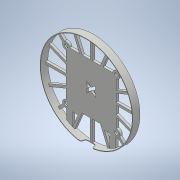
# Autodesk Inventor part: Чаша1
Saved by Autodesk Inventor 2020 (Build 240168000, 168)
## iProperties
Created: 2021-05-28
Part Number: Чаша1
Material: Типовые
Document SubType Name: Modeling
Designer: I_Love_U_Bogdan
Density: 1 g/cm^3
Appearance: По умолчанию
Author: I_Love_U_Bogdan
Autodesk Inventor part; units mm, degrees
ref_plane "YZ Plane" through (0, 0, 0) normal (1, 0, 0) x (0, 1, 0)
ref_plane "XZ Plane" through (0, 0, 0) normal (0, 1, 0) x (-1, 0, 0)
ref_plane "XY Plane" through (0, 0, 0) normal (0, 0, 1) x (1, 0, 0)
sketch "Эскиз1" plane through (0, 0, 0) normal (0, 0, 1) x (1, 0, 0)
  line L0 (7.05, 4.17398) -> (7.05, 6.642805)
  line L1 (7.05, 6.642805) -> (-5.95, -2.765587)
  line L2 (-5.95, -2.765587) -> (-5.95, 18.64843)
  line L3 (-5.95, 18.64843) -> (7.05, 9.240038)
  line L4 (7.05, 9.240038) -> (7.05, 11.708863)
  line L5 (7.05, 11.708863) -> (-4.244357, 19.882843)
  line L6 (-4.244357, 19.882843) -> (25.344357, 19.882843)
  line L7 (14.05, 11.708863) -> (25.344357, 19.882843)
  line L8 (14.05, 11.708863) -> (14.05, 9.240038)
  line L9 (27.05, 18.64843) -> (14.05, 9.240038)
  line L10 (27.05, -2.765587) -> (27.05, 18.64843)
  line L11 (14.05, 6.642805) -> (27.05, -2.765587)
  line L12 (14.05, 6.642805) -> (14.05, 4.17398)
  line L13 (25.344357, -4) -> (14.05, 4.17398)
  line L14 (-4.244357, -4) -> (25.344357, -4)
  line L15 (-4.244357, -4) -> (7.05, 4.17398)
  line L16 (-5.95, -6) -> (27.05, -6)
  line L17 (27.05, -32) -> (27.05, -6)
  line L18 (29.55, -33.117157) -> (29.55, -35)
  line L19 (31.65, -33.117157) -> (29.55, -33.117157)
  line L20 (31.65, -31.117157) -> (31.65, -33.117157)
  line L21 (29.55, -31.117157) -> (31.65, -31.117157)
  line L22 (29.55, -20.7) -> (29.55, -31.117157)
  line L23 (31.55, -20.7) -> (29.55, -20.7)
  line L24 (31.55, -19.7) -> (31.55, -20.7)
  line L25 (29.55, -16.235898) -> (31.55, -19.7)
  line L26 (29.55, 32) -> (29.55, 21.882843)
  line L27 (31.55, 19.882843) -> (29.55, 19.882843)
  line L28 (31.55, 19.882843) -> (31.55, 21.882843)
  line L29 (29.55, 21.882843) -> (31.55, 21.882843)
  line L30 (29.55, 32) -> (27.05, 32)
  line L31 (27.05, 21.882843) -> (27.05, 32)
  line L32 (-5.95, 21.882843) -> (27.05, 21.882843)
  line L33 (-5.95, 21.882843) -> (-5.95, 32)
  line L34 (-8.45, 32) -> (-5.95, 32)
  line L35 (-8.45, 32) -> (-8.45, 21.882843)
  line L36 (-8.45, 21.882843) -> (-10.45, 21.882843)
  line L37 (-10.45, 19.882843) -> (-10.45, 21.882843)
  line L38 (-10.45, 19.882843) -> (-8.45, 19.882843)
  line L39 (-8.45, -20.7) -> (-8.45, -31.117157)
  line L40 (-8.45, -16.235898) -> (-10.45, -19.7)
  line L41 (-10.45, -19.7) -> (-10.45, -20.7)
  line L42 (-10.45, -20.7) -> (-8.45, -20.7)
  line L43 (-8.45, -31.117157) -> (-10.55, -31.117157)
  line L44 (-10.55, -31.117157) -> (-10.55, -33.117157)
  line L45 (-10.55, -33.117157) -> (-8.45, -33.117157)
  line L46 (-8.45, -33.117157) -> (-8.45, -35)
  line L47 (-5.95, -32) -> (-5.95, -6)
  line L48 (10.55, 6.707009) -> (10.55, 9.175834)
  circle A0 centre (10.55, 7.941421) radius 38.2
  circle A1 centre (10.55, 7.941421) radius 38.7
  line L49 (27.05, -32) -> (27.026915, -32)
  line L50 (27.026915, -35) -> (27.026915, -32)
  line L51 (27.026915, -35) -> (29.55, -35)
  line L52 (29.55, 19.882843) -> (29.55, -16.235898)
  line L53 (-8.45, 19.882843) -> (-8.45, -16.235898)
  line L54 (-5.926915, -35) -> (-8.45, -35)
  line L55 (-5.926915, -35) -> (-5.926915, -32)
  line L56 (-5.95, -32) -> (-5.926915, -32)
  line L57 (13.55, 6.38746) -> (13.55, 5.153048)
  line L58 (11.402822, 7.941421) -> (13.55, 6.38746)
  line L59 (13.55, 9.495383) -> (11.402822, 7.941421)
  line L60 (13.55, 10.729795) -> (13.55, 9.495383)
  line L61 (10.55, 8.558628) -> (13.55, 10.729795)
  line L62 (7.55, 10.729795) -> (10.55, 8.558628)
  line L63 (7.55, 9.495383) -> (7.55, 10.729795)
  line L64 (9.697178, 7.941421) -> (7.55, 9.495383)
  line L65 (7.55, 6.38746) -> (9.697178, 7.941421)
  line L66 (7.55, 5.153048) -> (7.55, 6.38746)
  line L67 (10.55, 7.324215) -> (7.55, 5.153048)
  line L68 (13.55, 5.153048) -> (10.55, 7.324215)
  line L69 (-10.45, 28.941421) -> (31.55, 28.941421)
  line L70 (31.55, 28.941421) -> (31.55, -13.058579)
  line L71 (31.55, -13.058579) -> (-10.45, -13.058579)
  line L72 (-10.45, -13.058579) -> (-10.45, 28.941421)
  line L73 (-10.45, 28.941421) -> (31.55, -13.058579) construction
  line L74 (31.55, 28.941421) -> (-10.45, -13.058579) construction
  circle A2 centre (31.55, 28.941421) radius 1.5
  circle A3 centre (31.55, -13.058579) radius 1.5
  circle A4 centre (-10.45, -13.058579) radius 1.5
  circle A5 centre (-10.45, -13.058579) radius 3
  circle A6 centre (31.55, -13.058579) radius 3
  circle A7 centre (31.55, 28.941421) radius 3
  line L75 (34.55, 28.941421) -> (34.55, -13.058579)
  line L76 (31.55, -16.058579) -> (-10.45, -16.058579)
  line L77 (-13.45, -13.058579) -> (-13.45, 29.004231)
  line L78 (-10.391298, 31.941421) -> (31.55, 31.941421)
  circle A8 centre (-10.45, 28.941421) radius 1.5
  circle A9 centre (-10.45, 28.941421) radius 3
  line L79 (6.85, 9.1379) -> (6.85, 12.10049)
  line L80 (6.85, 12.10049) -> (10.55, 9.422716)
  line L81 (10.55, 9.422716) -> (14.25, 12.10049)
  line L82 (14.25, 12.10049) -> (14.25, 9.1379)
  line L83 (14.25, 9.1379) -> (12.596772, 7.941421)
  line L84 (12.596772, 7.941421) -> (14.25, 6.744943)
  line L85 (14.25, 6.744943) -> (14.25, 3.782353)
  line L86 (14.25, 3.782353) -> (10.55, 6.460126)
  line L87 (10.55, 6.460126) -> (6.85, 3.782353)
  line L88 (6.85, 3.782353) -> (6.85, 6.744943)
  line L89 (6.85, 6.744943) -> (8.503228, 7.941421)
  line L90 (8.503228, 7.941421) -> (6.85, 9.1379)
  line L91 (10.55, 7.941421) -> (10.55, 46.141421) construction
  line L92 (11.55, 28.941421) -> (11.55, 46.141421)
  line L93 (9.55, 46.141421) -> (9.55, 28.941421)
  line L94 (9.55, 9.28235) -> (9.55, 8.941421)
  line L95 (9.55, 8.047938) -> (9.55, 7.941421)
  line L96 (11.55, 7.941421) -> (11.55, 8.047938)
  line L97 (11.55, 8.941421) -> (11.55, 9.28235)
  line L98 (3.437527, 27.725575) -> (-3.144628, 43.616303)
  line L99 (-4.992387, 42.850936) -> (1.589768, 26.960208)
  line L100 (-3.592136, 23.497771) -> (-15.754372, 35.660007)
  line L101 (-17.168586, 34.245794) -> (-5.006349, 22.083557)
  line L102 (-8.468787, 16.901653) -> (-24.359515, 23.483808)
  line L103 (-25.124882, 21.636049) -> (-9.234154, 15.053894)
  line L104 (-10.45, 8.941421) -> (-27.65, 8.941421)
  line L105 (-27.65, 6.941421) -> (-10.45, 6.941421)
  line L106 (-9.234154, 0.828949) -> (-25.124882, -5.753206)
  line L107 (-24.359515, -7.600965) -> (-8.468787, -1.01881)
  line L108 (-5.006349, -6.200714) -> (-17.168586, -18.362951)
  line L109 (-15.754372, -19.777164) -> (-3.592136, -7.614928)
  line L110 (1.589768, -11.077365) -> (-4.992387, -26.968093)
  line L111 (-3.144628, -27.73346) -> (3.437527, -11.842732)
  line L112 (9.55, -13.058579) -> (9.55, -30.258579)
  line L113 (11.55, -30.258579) -> (11.55, -13.058579)
  line L114 (17.662473, -11.842732) -> (24.244628, -27.73346)
  line L115 (26.092387, -26.968093) -> (19.510232, -11.077365)
  line L116 (24.692136, -7.614928) -> (36.854372, -19.777164)
  line L117 (38.268586, -18.362951) -> (26.106349, -6.200714)
  line L118 (29.568787, -1.01881) -> (45.459515, -7.600965)
  line L119 (46.224882, -5.753206) -> (30.334154, 0.828949)
  line L120 (31.55, 6.941421) -> (48.75, 6.941421)
  line L121 (48.75, 8.941421) -> (31.55, 8.941421)
  line L122 (30.334154, 15.053894) -> (46.224882, 21.636049)
  line L123 (45.459515, 23.483808) -> (29.568787, 16.901653)
  line L124 (26.106349, 22.083557) -> (38.268586, 34.245794)
  line L125 (36.854372, 35.660007) -> (24.692136, 23.497771)
  line L126 (19.510232, 26.960208) -> (26.092387, 42.850936)
  line L127 (24.244628, 43.616303) -> (17.662473, 27.725575)
  line L128 (-4.992387, -16.058579) -> (-9.992387, -16.058579)
  line L129 (-9.992387, -16.058579) -> (-9.992387, -24.85645)
  line L130 (-9.992387, -27.058579) -> (-4.992387, -27.058579)
  line L131 (-4.992387, -27.058579) -> (-4.992387, -16.058579)
  line L132 (31.092387, -16.058579) -> (31.092387, -24.85645)
  line L133 (26.092387, -27.058579) -> (26.092387, -16.058579)
  point P0 (0, 0)
  point P1 (10.55, 27.041421)
  point P2 (-10.45, 15.557514)
  point P3 (-27.636909, 8.941421)
  point P4 (-25.112787, 21.631039)
  point P5 (2.933907, 28.941421)
  point P6 (-3.139618, 43.604208)
  point P7 (9.55, 46.12833)
  point P8 (34.257107, -14.351472)
  point P9 (31.55, -10.058579)
  point P10 (31.55, -1.839456)
  point P11 (45.44742, -7.595955)
  point P12 (38.259329, -18.353694)
  point P13 (0.769123, 28.941421)
  point P14 (-7.45, 28.941421)
  point P15 (-11.742893, 31.648528)
  point P16 (-15.745115, 35.65075)
  point P17 (-4.987377, 42.838841)
  point P18 (-10.45, 17.722298)
  point P19 (-24.34742, 23.478798)
  point P20 (-17.159329, 34.236537)
  point P21 (-13.157107, 30.234315)
  point P22 (-10.45, 25.941421)
  point P23 (-0.473518, -16.058579)
  point P24 (2.933907, -13.058579)
  point P25 (9.55, -30.245487)
  point P26 (-3.139618, -27.721365)
  point P27 (18.166093, -13.058579)
  point P28 (24.239618, -27.721365)
  point P29 (11.55, -30.245487)
  point P30 (21.573518, -16.058579)
  point P31 (32.842893, 31.648528)
  point P32 (28.55, 28.941421)
  point P33 (20.330877, 28.941421)
  point P34 (26.087377, 42.838841)
  point P35 (36.845115, 35.65075)
  point P36 (31.55, 17.722298)
  point P37 (31.55, 25.941421)
  point P38 (34.257107, 30.234315)
  point P39 (38.259329, 34.236537)
  point P40 (45.44742, 23.478798)
  point P41 (31.55, 15.557514)
  point P42 (46.212787, 21.631039)
  point P43 (48.736909, 8.941421)
  point P44 (31.55, 0.325329)
  point P45 (48.736909, 6.941421)
  point P46 (46.212787, -5.748196)
  point P47 (32.842893, -15.765685)
  point P48 (36.845115, -19.767908)
  point P49 (31.092387, -24.26495)
  point P50 (-5.963328, -27.058579)
  point P51 (-5.95, -27.058579)
  point P52 (-5.95, -27.064864)
  point P53 (-11.742893, -15.765685)
  point P54 (-9.992387, -24.26495)
  point P55 (-15.745115, -19.767908)
  point P56 (-10.45, -1.839456)
  point P57 (-10.45, -10.058579)
  point P58 (-13.157107, -14.351472)
  point P59 (-17.159329, -18.353694)
  point P60 (-24.34742, -7.595955)
  point P61 (-10.45, 0.325329)
  point P62 (-25.112787, -5.748196)
  point P63 (-27.636909, 6.941421)
  point P64 (11.55, 46.12833)
  point P65 (24.239618, 43.604208)
  point P66 (18.166093, 28.941421)
  dimension "d0" = 76.4
  dimension "d1" = 0.5
  dimension "d15" = 42
  dimension "d16" = 42
  dimension "d17" = 3
  dimension "d18" = 3
  dimension "d19" = 3
  dimension "d22" = 6
  dimension "d23" = 6
  dimension "d24" = 6
  dimension "d25" = 3
  dimension "d26" = 1.5
  dimension "d27" = 0.7
  dimension "d31" = 360
  dimension "d33" = 5
  dimension "d34" = 11
  constraints: 134 end point, 13 parallel, 9 point on line, 8 centre point, 8 coincident, 7 tangent, 6 point on circle, 4 midpoint, 4 symmetric about line, 3 perpendicular, 2 horizontal, 2 vertical, 114 other
  measures "d15" distance of L70.end L71.end
  measures "d16" distance of L69.end L70.end
  measures "d17" diameter of A2
  measures "d18" diameter of A3
  measures "d19" diameter of A4
  measures "d22" diameter of A5
  measures "d23" diameter of A6
  measures "d24" diameter of A7
  measures "d25" diameter of A8
  measures "d26" radial gap between concentric circles of A8 A9
  measures "d27" distance between parallel lines of L64 L90
  measures "d33" distance of L130.end L130.start
  measures "d34" distance of L130.start L128.end
sketch "Эскиз1 outline for Выдавливание1" plane through (0, 0, 0) normal (0, 0, 1) x (1, 0, 0)
  arc A0 (-5.95, -27.064864) -> (-5.963328, -27.058579) centre (10.55, 7.941421) ccw
  arc A1 (-5.963328, -27.058579) -> (-5.95, -27.064864) centre (10.55, 7.941421) ccw
  arc A2 (-11.742893, -15.765685) -> (-10.45, -16.058579) centre (-10.45, -13.058579) ccw
  line L0 (-10.45, -16.058579) -> (-9.992387, -16.058579)
  line L1 (-9.992387, -16.058579) -> (-9.992387, -24.26495)
  arc A3 (-9.992387, -24.26495) -> (-15.745115, -19.767908) centre (10.55, 7.941421) cw
  line L2 (-15.745115, -19.767908) -> (-11.742893, -15.765685)
  circle A4 centre (-10.45, -13.058579) radius 1.5
  line L3 (-4.992387, -26.968093) -> (-4.992387, -16.058579)
  line L4 (-4.992387, -16.058579) -> (-0.473518, -16.058579)
  line L5 (-0.473518, -16.058579) -> (-4.992387, -26.968093)
  line L6 (-3.139618, -27.721365) -> (2.933907, -13.058579)
  line L7 (2.933907, -13.058579) -> (9.55, -13.058579)
  line L8 (9.55, -13.058579) -> (9.55, -30.245487)
  arc A5 (9.55, -30.245487) -> (-3.139618, -27.721365) centre (10.55, 7.941421) cw
  line L9 (-24.34742, -7.595955) -> (-10.45, -1.839456)
  line L10 (-10.45, -1.839456) -> (-10.45, -10.058579)
  arc A6 (-10.45, -10.058579) -> (-13.157107, -14.351472) centre (-10.45, -13.058579) ccw
  line L11 (-13.157107, -14.351472) -> (-17.159329, -18.353694)
  arc A7 (-17.159329, -18.353694) -> (-24.34742, -7.595955) centre (10.55, 7.941421) cw
  line L12 (-27.636909, 6.941421) -> (-10.45, 6.941421)
  line L13 (-10.45, 6.941421) -> (-10.45, 0.325329)
  line L14 (-10.45, 0.325329) -> (-25.112787, -5.748196)
  arc A8 (-25.112787, -5.748196) -> (-27.636909, 6.941421) centre (10.55, 7.941421) cw
  line L15 (6.85, 3.782353) -> (6.85, 6.744943)
  line L16 (6.85, 6.744943) -> (8.503228, 7.941421)
  line L17 (8.503228, 7.941421) -> (6.85, 9.1379)
  line L18 (6.85, 9.1379) -> (6.85, 12.10049)
  line L19 (6.85, 12.10049) -> (10.55, 9.422716)
  line L20 (10.55, 9.422716) -> (14.25, 12.10049)
  line L21 (14.25, 12.10049) -> (14.25, 9.1379)
  line L22 (14.25, 9.1379) -> (12.596772, 7.941421)
  line L23 (12.596772, 7.941421) -> (14.25, 6.744943)
  line L24 (14.25, 6.744943) -> (14.25, 3.782353)
  line L25 (14.25, 3.782353) -> (10.55, 6.460126)
  line L26 (10.55, 6.460126) -> (6.85, 3.782353)
  line L27 (11.55, -30.245487) -> (11.55, -13.058579)
  line L28 (11.55, -13.058579) -> (18.166093, -13.058579)
  line L29 (18.166093, -13.058579) -> (24.239618, -27.721365)
  arc A9 (24.239618, -27.721365) -> (11.55, -30.245487) centre (10.55, 7.941421) cw
  line L30 (21.573518, -16.058579) -> (26.092387, -16.058579)
  line L31 (26.092387, -16.058579) -> (26.092387, -26.968093)
  line L32 (26.092387, -26.968093) -> (21.573518, -16.058579)
  line L33 (32.842893, -15.765685) -> (36.845115, -19.767908)
  arc A10 (36.845115, -19.767908) -> (31.092387, -24.26495) centre (10.55, 7.941421) cw
  line L34 (31.092387, -24.26495) -> (31.092387, -16.058579)
  line L35 (31.092387, -16.058579) -> (31.55, -16.058579)
  arc A11 (31.55, -16.058579) -> (32.842893, -15.765685) centre (31.55, -13.058579) ccw
  circle A12 centre (31.55, -13.058579) radius 1.5
  arc A13 (34.257107, -14.351472) -> (31.55, -10.058579) centre (31.55, -13.058579) ccw
  line L36 (31.55, -10.058579) -> (31.55, -1.839456)
  line L37 (31.55, -1.839456) -> (45.44742, -7.595955)
  arc A14 (45.44742, -7.595955) -> (38.259329, -18.353694) centre (10.55, 7.941421) cw
  line L38 (38.259329, -18.353694) -> (34.257107, -14.351472)
  line L39 (46.212787, -5.748196) -> (31.55, 0.325329)
  line L40 (31.55, 0.325329) -> (31.55, 6.941421)
  line L41 (31.55, 6.941421) -> (48.736909, 6.941421)
  arc A15 (48.736909, 6.941421) -> (46.212787, -5.748196) centre (10.55, 7.941421) cw
  line L42 (-10.45, 15.557514) -> (-10.45, 8.941421)
  line L43 (-10.45, 8.941421) -> (-27.636909, 8.941421)
  arc A16 (-27.636909, 8.941421) -> (-25.112787, 21.631039) centre (10.55, 7.941421) cw
  line L44 (-25.112787, 21.631039) -> (-10.45, 15.557514)
  line L45 (-10.45, 17.722298) -> (-24.34742, 23.478798)
  arc A17 (-24.34742, 23.478798) -> (-17.159329, 34.236537) centre (10.55, 7.941421) cw
  line L46 (-17.159329, 34.236537) -> (-13.157107, 30.234315)
  arc A18 (-13.157107, 30.234315) -> (-10.45, 25.941421) centre (-10.45, 28.941421) ccw
  line L47 (-10.45, 25.941421) -> (-10.45, 17.722298)
  circle A19 centre (-10.45, 28.941421) radius 1.5
  line L48 (-4.987377, 42.838841) -> (0.769123, 28.941421)
  line L49 (0.769123, 28.941421) -> (-7.45, 28.941421)
  arc A20 (-7.45, 28.941421) -> (-11.742893, 31.648528) centre (-10.45, 28.941421) ccw
  line L50 (-11.742893, 31.648528) -> (-15.745115, 35.65075)
  arc A21 (-15.745115, 35.65075) -> (-4.987377, 42.838841) centre (10.55, 7.941421) cw
  line L51 (9.55, 46.12833) -> (9.55, 28.941421)
  line L52 (9.55, 28.941421) -> (2.933907, 28.941421)
  line L53 (2.933907, 28.941421) -> (-3.139618, 43.604208)
  arc A22 (-3.139618, 43.604208) -> (9.55, 46.12833) centre (10.55, 7.941421) cw
  line L54 (48.736909, 8.941421) -> (31.55, 8.941421)
  line L55 (31.55, 8.941421) -> (31.55, 15.557514)
  line L56 (31.55, 15.557514) -> (46.212787, 21.631039)
  arc A23 (46.212787, 21.631039) -> (48.736909, 8.941421) centre (10.55, 7.941421) cw
  line L57 (45.44742, 23.478798) -> (31.55, 17.722298)
  line L58 (31.55, 17.722298) -> (31.55, 25.941421)
  arc A24 (31.55, 25.941421) -> (34.257107, 30.234315) centre (31.55, 28.941421) ccw
  line L59 (34.257107, 30.234315) -> (38.259329, 34.236537)
  arc A25 (38.259329, 34.236537) -> (45.44742, 23.478798) centre (10.55, 7.941421) cw
  arc A26 (32.842893, 31.648528) -> (28.55, 28.941421) centre (31.55, 28.941421) ccw
  line L60 (28.55, 28.941421) -> (20.330877, 28.941421)
  line L61 (20.330877, 28.941421) -> (26.087377, 42.838841)
  arc A27 (26.087377, 42.838841) -> (36.845115, 35.65075) centre (10.55, 7.941421) cw
  line L62 (36.845115, 35.65075) -> (32.842893, 31.648528)
  line L63 (11.55, 28.941421) -> (11.55, 46.12833)
  arc A28 (11.55, 46.12833) -> (24.239618, 43.604208) centre (10.55, 7.941421) cw
  line L64 (24.239618, 43.604208) -> (18.166093, 28.941421)
  line L65 (18.166093, 28.941421) -> (11.55, 28.941421)
  circle A29 centre (31.55, 28.941421) radius 1.5
extrude "Выдавливание1" add sketch "Эскиз1 outline for Выдавливание1" along normal blind 2
chamfer "Фаска2" distance 0.5 angle 45 12 edges at (8.7, 10.7616, 0) (12.4, 10.7616, 0) (13.4234, 8.5397, 0) (13.4234, 7.3432, 0) (14.25, 5.2636, 0) (12.4, 5.1212, 0) (8.7, 5.1212, 0) (6.85, 5.2636, 0) (7.6766, 7.3432, 0) (7.6766, 8.5397, 0) (6.85, 10.6192, 0) (14.25, 10.6192, 0)
chamfer "Фаска3" distance 1 angle 45 4 edges at (30.05, 28.9414, 0) (-11.95, 28.9414, 0) (-11.95, -13.0586, 0) (30.05, -13.0586, 0)
sketch "Эскиз4" plane through (0, 0, 2) normal (0, 0, 1) x (1, 0, 0)
  circle A0 centre (10.55, 7.941421) radius 38.7
  circle A1 centre (10.55, 7.941421) radius 38.2
  line L0 (15.05, -33.04811) -> (6.05, -33.04811)
  line L1 (6.05, 48.930952) -> (15.05, -33.04811) construction
  line L2 (15.05, 48.930952) -> (6.05, -33.04811) construction
  line L3 (6.05, -30.49606) -> (6.05, -29.9926)
  line L4 (15.05, -29.9926) -> (15.05, -30.49606)
  circle A2 centre (10.55, 7.941421) radius 38.7
  point P0 (0, 0)
  point P1 (-5.95, -27.064864)
  point P2 (-5.963328, -27.058579)
  point P3 (-5.963328, -27.058579)
  point P4 (-5.95, -27.064864)
  dimension "d41" = 0.5
  dimension "d42" = 9
  constraints: 10 end point, 4 point on circle, 2 centre point, 2 coincident, 2 midpoint, 1 parallel
  measures "d41" radial gap between concentric circles of A0 A1
  measures "d42" distance of L0.start L0.end
extrude "Выдавливание4" add sketch "Эскиз4" along normal blind 4 contours A0 L4 A1 L3 picked at (48.472124, 13.505691)
fillet "Сопряжение2" radius 2 4 edges at (15.05, -30.2443, 6) (6.05, -30.2443, 6) (6.05, -30.2443, 2) (15.05, -30.2443, 2)
